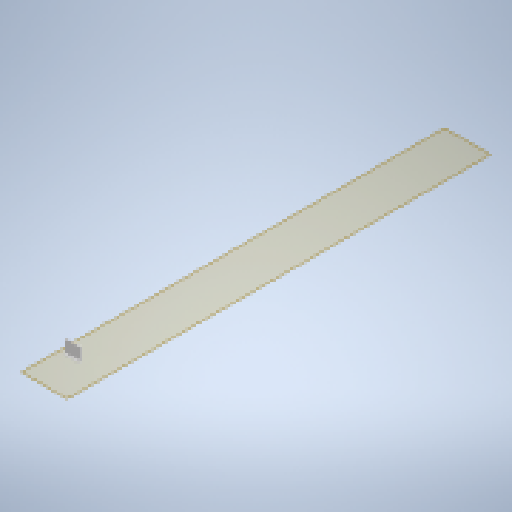
# Autodesk Inventor part: backCase
Saved by Autodesk Inventor 2023 (Build 270158000, 158)
## iProperties
Created: 2022-12-09
Part Number: backCase
Material: Generic
Document SubType Name: Modeling
Designer: shrey
Density: 1 g/cm^3
Appearance: Default
Author: shrey
Autodesk Inventor part; units mm, degrees
ref_plane "YZ Plane" through (0, 0, 0) normal (1, 0, 0) x (0, 1, 0)
ref_plane "XZ Plane" through (0, 0, 0) normal (0, 1, 0) x (-1, 0, 0)
ref_plane "XY Plane" through (0, 0, 0) normal (0, 0, 1) x (1, 0, 0)
ref_plane "Work Plane1" through (88.0411, 0, -4.3553) normal (0, 1, 0) x (-1, 0, 0)
sketch "Sketch1" plane through (88.0411, 0, -4.3553) normal (0, 1, 0) x (-1, 0, 0)
  line L0 (58.171, -0.729) -> (56.0977, -0.729) projected
  line L1 (56.0977, -0.729) -> (54.0127, -0.3924) projected
  line L2 (54.0127, -0.3924) -> (50.0902, -0.0001) projected
  line L3 (50.0902, -0.0001) -> (48.159, -0.0001) projected
  line L4 (48.159, -0.0001) -> (48.159, -0.9194) projected
  line L5 (48.159, -0.9194) -> (46.281, -0.9194) projected
  line L6 (46.281, -0.9194) -> (44.3734, -0.6114) projected
  line L7 (44.3734, -0.6114) -> (42.5702, -0.4904) projected
  line L8 (42.5702, -0.4904) -> (38.7992, -0.4904) projected
  line L9 (38.7992, -0.4904) -> (36.9307, -0.729) projected
  line L10 (36.9307, -0.729) -> (35.0405, -1.2743) projected
  line L11 (35.0405, -1.2743) -> (32.7869, -1.7551) projected
  line L12 (32.7869, -1.7551) -> (31.1597, -2.2246) projected
  line L13 (31.1597, -2.2246) -> (29.2392, -2.5119) projected
  line L14 (29.2392, -2.5119) -> (25.7568, -2.5119) projected
  line L15 (25.7568, -2.5119) -> (22.1476, -1.9292) projected
  line L16 (22.1476, -1.9292) -> (20.1771, -1.9292) projected
  line L17 (20.1771, -1.9292) -> (20.1771, -3.0939) projected
  line L18 (20.1771, -3.0939) -> (15.2755, -3.0939) projected
  line L19 (15.2755, -3.0939) -> (12.2384, -2.6036) projected
  line L20 (12.2384, -2.6036) -> (10.4528, -2.6036) projected
  line L21 (10.4528, -2.6036) -> (8.2143, -2.8887) projected
  line L22 (8.2143, -2.8887) -> (6.4213, -2.7683) projected
  line L23 (6.4213, -2.7683) -> (6.4213, -2.4041) projected
  line L24 (6.4213, -2.4041) -> (3.9663, -2.6036) projected
  line L25 (3.9663, -2.6036) -> (1.931, -2.8628) projected
  line L26 (1.931, -2.8628) -> (-0.0002, -2.7332) projected
  line L27 (-0.0002, -2.7332) -> (-0.0002, -9.8132) projected
  line L28 (-0.0002, -9.8132) -> (-6.1102, -9.8132) projected
  line L29 (-6.1102, -9.8132) -> (-6.1102, -18.749) projected
  line L30 (-6.1102, -18.749) -> (58.171, -18.749) projected
  line L31 (58.171, -18.749) -> (58.171, -0.729) projected
  line L32 (58.171, -0.0001) -> (-0.0002, -0.0001)
  line L33 (-0.0002, -0.0001) -> (-0.0002, -2.7332)
  line L34 (-0.0002, -2.7332) -> (58.171, -2.7332)
  line L35 (58.171, -2.7332) -> (58.171, -0.0001)
  line L36 (-0.0002, -0.0001) -> (81.9998, -0.0001)
  line L37 (81.9998, -0.0001) -> (81.9998, 1.9999)
  line L38 (81.9998, 1.9999) -> (-0.0002, 1.9999)
  line L39 (-0.0002, 1.9999) -> (-0.0002, -0.0001)
  point P0 (88.0411, 4.3553)
  point P1 (2.9486, -2.7332)
  point P2 (6.4213, -2.7332)
  point P3 (9.4352, -2.7332)
  point P4 (31.9998, 9.1499)
  point P5 (20.1771, -2.7332)
  point P6 (13.0411, -2.7332)
  point P7 (48.159, -0.0001)
  point P8 (58.171, -2.7332)
  point P9 (50.0902, -0.0001)
  dimension "d0" = 2
  dimension "d13" = 50
  constraints: 16 end point, 4 parallel, 3 horizontal, 2 perpendicular, 1 point on line
  measures "d0" distance of L37.end L36.end
  measures "d13" distance from line of point (32, 9.15) L37
extrude "Extrusion1" add sketch "Sketch1" along normal blind 50 contours L31 L34 L17 L16 L15 L14 L13 L12 L11 L10 L9 L8 L7 L6 L5 L4 L3 L2 L1 L0 | L0 L1 L2 L32 L35 | L32 L3 L39 L38 L37 L36 | L34 L19 L20 L21 L23 L24 L25 L33 L32 L4 L5 L6 L7 L8 L9 L10 L11 L12 L13 L14 L15 L16 L17 | L34 L21 L20 L19 | L21 L22 L23 L34 | L34 L25 L24 L23 | L34 L25 L26
sketch "Sketch2" plane through (6.0413, 0, -2.3554) normal (0, 0, 1) x (1, 0, 0)
  line L0 (2.0733, 0) -> (0, 0) projected
  line L1 (82, 0) -> (82, 50) projected
  line L2 (0, 0) -> (82, 0)
  line L3 (82, 0) -> (82, 3)
  line L4 (82, 3) -> (0, 3)
  line L5 (0, 3) -> (0, 0)
  circle A0 centre (50, 40.5) radius 32 construction
  line L6 (58.1712, -304.8) -> (58.1712, 304.8) construction
  circle A1 centre (50, 40.5) radius 3.925
  circle A2 centre (50, 40.5) radius 1.925
  point P0 (-6.0413, 0)
  point P1 (10, 40.5)
  dimension "d3" = 3
  dimension "d6" = 64
  dimension "d7" = 37.5
  dimension "d8" = 32
  dimension "d9" = 7.85
  dimension "d10" = 2
  dimension "d14" = 40
  constraints: 8 end point, 3 centre point, 2 parallel, 1 coincident, 1 horizontal, 1 perpendicular, 1 point on line, 1 other
  measures "d3" distance of L3.end L2.end
  measures "d6" diameter of A0
  measures "d7" distance from line of L4 A0.centre
  measures "d8" distance from line of L1 A0.centre
  measures "d9" diameter of A1
  measures "d10" radial gap between concentric circles of A1 A2
  measures "d14" distance of point (10, 40.5) A0.centre
extrude "Extrusion2" add sketch "Sketch2" along normal blind 7 contours L0 L5 L4 L1 L2
extrude "Extrusion3" add sketch "Sketch2" along normal blind 7.15 contours A1
equation "\"t\" = 0.15"
body "Solid1"
